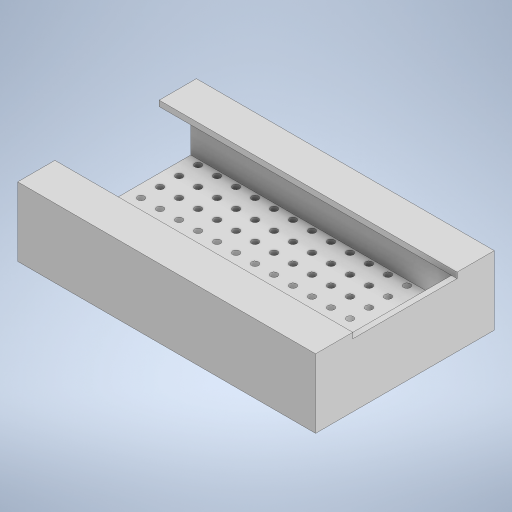
# Autodesk Inventor part: support batterie
Saved by Autodesk Inventor 2024 (Build 280153000, 153)
## iProperties
Created: 2024-02-10
Part Number: support batterie
Material: Generic
Document SubType Name: Modeling
Designer: Pooo
Density: 1 g/cm^3
Appearance: Default
Author: Pooo
Autodesk Inventor part; units mm, degrees
ref_plane "YZ Plane" through (0, 0, 0) normal (1, 0, 0) x (0, 1, 0)
ref_plane "XZ Plane" through (0, 0, 0) normal (0, 1, 0) x (-1, 0, 0)
ref_plane "XY Plane" through (0, 0, 0) normal (0, 0, 1) x (1, 0, 0)
sketch "Sketch1" plane through (0, 0, 0) normal (0, 1, 0) x (-1, 0, 0)
  point P0 (0, 0)
sketch "Sketch2" plane through (0, 0, 0) normal (0, 1, 0) x (-1, 0, 0)
  line L0 (43.1586, 43.7586) -> (-113.8414, 43.7586)
  line L1 (-113.8414, 43.7586) -> (-113.8414, -46.2414)
  line L2 (-113.8414, -46.2414) -> (43.1586, -46.2414)
  line L3 (43.1586, -46.2414) -> (43.1586, 43.7586)
  line L4 (43.1586, -46.2414) -> (-113.8414, -46.2414)
  line L5 (-113.8414, -46.2414) -> (-113.8414, -49.2414)
  line L6 (-113.8414, -49.2414) -> (43.1586, -49.2414)
  line L7 (43.1586, -49.2414) -> (43.1586, -46.2414)
  line L8 (43.1586, 43.7586) -> (-113.8414, 43.7586)
  line L9 (-113.8414, 43.7586) -> (-113.8414, 46.7586)
  line L10 (-113.8414, 46.7586) -> (43.1586, 46.7586)
  line L11 (43.1586, 46.7586) -> (43.1586, 43.7586)
  line L12 (-113.8414, 46.7586) -> (-116.8414, 46.7586)
  line L13 (-116.8414, 46.7586) -> (-116.8414, -49.2414)
  line L14 (-116.8414, -49.2414) -> (-113.8414, -49.2414)
  line L15 (-113.8414, -49.2414) -> (-113.8414, 46.7586)
  point P0 (0, 0)
  dimension "d0" = 90
  dimension "d1" = 157
  dimension "d2" = 3
  dimension "d3" = 3
  dimension "d4" = 3
  constraints: 32 end point, 8 parallel, 4 horizontal, 4 perpendicular
  measures "d0" distance of L2.end L0.start
  measures "d1" distance of L1.end L2.end
  measures "d2" distance of L4.end L5.end
  measures "d3" distance of L8.end L9.end
  measures "d4" distance of L14.end L13.end
extrude "Extrusion1" add sketch "Sketch2" along normal blind 3
sketch "Sketch3" plane through (0, 3, 0) normal (0, 1, 0) x (1, 0, 0)
  line L0 (-43.1586, -46.7586) -> (116.8414, -46.7586) projected
  line L1 (116.8414, -46.7586) -> (116.8414, 49.2414) projected
  line L2 (-43.1586, -46.7586) -> (116.8414, -46.7586)
  line L3 (116.8414, -46.7586) -> (116.8414, -43.7586)
  line L4 (116.8414, -43.7586) -> (-43.1586, -43.7586)
  line L5 (-43.1586, -43.7586) -> (-43.1586, -46.7586)
  line L6 (116.8414, 49.2414) -> (-43.1586, 49.2414) projected
  line L7 (-43.1586, 49.2414) -> (116.8414, 49.2414)
  line L8 (116.8414, 49.2414) -> (116.8414, 46.2414)
  line L9 (116.8414, 46.2414) -> (-43.1586, 46.2414)
  line L10 (-43.1586, 46.2414) -> (-43.1586, 49.2414)
  line L11 (116.8414, -43.7586) -> (113.8414, -43.7586)
  line L12 (113.8414, -43.7586) -> (113.8414, 46.2414)
  line L13 (113.8414, 46.2414) -> (116.8414, 46.2414)
  line L14 (116.8414, 46.2414) -> (116.8414, -43.7586)
  point P0 (0, 0)
  dimension "d7" = 3
  dimension "d8" = 3
  dimension "d9" = 3
  constraints: 24 end point, 6 parallel, 3 horizontal, 3 perpendicular, 3 point on line
  measures "d7" distance of L3.end L2.end
  measures "d8" distance of L7.end L8.end
  measures "d9" distance of L12.end L13.end
sketch "Sketch5" plane through (0, 3, 0) normal (0, 1, 0) x (1, 0, 0)
  circle A0 centre (-36.5125, -38.1) radius 1.85
  line L0 (-36.5125, -38.1) -> (-35.8777, -38.1)
  line L1 (-36.5125, -38.1) -> (-36.5125, -37.4601)
  circle A1 centre (-36.5125, -27.9) radius 1.85
  circle A2 centre (-36.5125, -17.7) radius 1.85
  circle A3 centre (-36.5125, -7.5) radius 1.85
  circle A4 centre (-36.5125, 2.7) radius 1.85
  circle A5 centre (-36.5125, 12.9) radius 1.85
  circle A6 centre (-36.5125, 23.1) radius 1.85
  circle A7 centre (-36.5125, 33.3) radius 1.85
  circle A8 centre (-36.5125, 43.5) radius 1.85
  circle A9 centre (-26.3125, -38.1) radius 1.85
  circle A10 centre (-26.3125, -27.9) radius 1.85
  circle A11 centre (-26.3125, -17.7) radius 1.85
  circle A12 centre (-26.3125, -7.5) radius 1.85
  circle A13 centre (-26.3125, 2.7) radius 1.85
  circle A14 centre (-26.3125, 12.9) radius 1.85
  circle A15 centre (-26.3125, 23.1) radius 1.85
  circle A16 centre (-26.3125, 33.3) radius 1.85
  circle A17 centre (-26.3125, 43.5) radius 1.85
  circle A18 centre (-16.1125, -38.1) radius 1.85
  circle A19 centre (-16.1125, -27.9) radius 1.85
  circle A20 centre (-16.1125, -17.7) radius 1.85
  circle A21 centre (-16.1125, -7.5) radius 1.85
  circle A22 centre (-16.1125, 2.7) radius 1.85
  circle A23 centre (-16.1125, 12.9) radius 1.85
  circle A24 centre (-16.1125, 23.1) radius 1.85
  circle A25 centre (-16.1125, 33.3) radius 1.85
  circle A26 centre (-16.1125, 43.5) radius 1.85
  circle A27 centre (-5.9125, -38.1) radius 1.85
  circle A28 centre (-5.9125, -27.9) radius 1.85
  circle A29 centre (-5.9125, -17.7) radius 1.85
  circle A30 centre (-5.9125, -7.5) radius 1.85
  circle A31 centre (-5.9125, 2.7) radius 1.85
  circle A32 centre (-5.9125, 12.9) radius 1.85
  circle A33 centre (-5.9125, 23.1) radius 1.85
  circle A34 centre (-5.9125, 33.3) radius 1.85
  circle A35 centre (-5.9125, 43.5) radius 1.85
  circle A36 centre (4.2875, -38.1) radius 1.85
  circle A37 centre (4.2875, -27.9) radius 1.85
  circle A38 centre (4.2875, -17.7) radius 1.85
  circle A39 centre (4.2875, -7.5) radius 1.85
  circle A40 centre (4.2875, 2.7) radius 1.85
  circle A41 centre (4.2875, 12.9) radius 1.85
  circle A42 centre (4.2875, 23.1) radius 1.85
  circle A43 centre (4.2875, 33.3) radius 1.85
  circle A44 centre (4.2875, 43.5) radius 1.85
  circle A45 centre (14.4875, -38.1) radius 1.85
  circle A46 centre (14.4875, -27.9) radius 1.85
  circle A47 centre (14.4875, -17.7) radius 1.85
  circle A48 centre (14.4875, -7.5) radius 1.85
  circle A49 centre (14.4875, 2.7) radius 1.85
  circle A50 centre (14.4875, 12.9) radius 1.85
  circle A51 centre (14.4875, 23.1) radius 1.85
  circle A52 centre (14.4875, 33.3) radius 1.85
  circle A53 centre (14.4875, 43.5) radius 1.85
  circle A54 centre (24.6875, -38.1) radius 1.85
  circle A55 centre (24.6875, -27.9) radius 1.85
  circle A56 centre (24.6875, -17.7) radius 1.85
  circle A57 centre (24.6875, -7.5) radius 1.85
  circle A58 centre (24.6875, 2.7) radius 1.85
  circle A59 centre (24.6875, 12.9) radius 1.85
  circle A60 centre (24.6875, 23.1) radius 1.85
  circle A61 centre (24.6875, 33.3) radius 1.85
  circle A62 centre (24.6875, 43.5) radius 1.85
  circle A63 centre (34.8875, -38.1) radius 1.85
  circle A64 centre (34.8875, -27.9) radius 1.85
  circle A65 centre (34.8875, -17.7) radius 1.85
  circle A66 centre (34.8875, -7.5) radius 1.85
  circle A67 centre (34.8875, 2.7) radius 1.85
  circle A68 centre (34.8875, 12.9) radius 1.85
  circle A69 centre (34.8875, 23.1) radius 1.85
  circle A70 centre (34.8875, 33.3) radius 1.85
  circle A71 centre (34.8875, 43.5) radius 1.85
  circle A72 centre (45.0875, -38.1) radius 1.85
  circle A73 centre (45.0875, -27.9) radius 1.85
  circle A74 centre (45.0875, -17.7) radius 1.85
  circle A75 centre (45.0875, -7.5) radius 1.85
  circle A76 centre (45.0875, 2.7) radius 1.85
  circle A77 centre (45.0875, 12.9) radius 1.85
  circle A78 centre (45.0875, 23.1) radius 1.85
  circle A79 centre (45.0875, 33.3) radius 1.85
  circle A80 centre (45.0875, 43.5) radius 1.85
  circle A81 centre (55.2875, -38.1) radius 1.85
  circle A82 centre (55.2875, -27.9) radius 1.85
  circle A83 centre (55.2875, -17.7) radius 1.85
  circle A84 centre (55.2875, -7.5) radius 1.85
  circle A85 centre (55.2875, 2.7) radius 1.85
  circle A86 centre (55.2875, 12.9) radius 1.85
  circle A87 centre (55.2875, 23.1) radius 1.85
  circle A88 centre (55.2875, 33.3) radius 1.85
  circle A89 centre (55.2875, 43.5) radius 1.85
  circle A90 centre (65.4875, -38.1) radius 1.85
  circle A91 centre (65.4875, -27.9) radius 1.85
  circle A92 centre (65.4875, -17.7) radius 1.85
  circle A93 centre (65.4875, -7.5) radius 1.85
  circle A94 centre (65.4875, 2.7) radius 1.85
  circle A95 centre (65.4875, 12.9) radius 1.85
  circle A96 centre (65.4875, 23.1) radius 1.85
  circle A97 centre (65.4875, 33.3) radius 1.85
  circle A98 centre (65.4875, 43.5) radius 1.85
  circle A99 centre (75.6875, -38.1) radius 1.85
  circle A100 centre (75.6875, -27.9) radius 1.85
  circle A101 centre (75.6875, -17.7) radius 1.85
  circle A102 centre (75.6875, -7.5) radius 1.85
  circle A103 centre (75.6875, 2.7) radius 1.85
  circle A104 centre (75.6875, 12.9) radius 1.85
  circle A105 centre (75.6875, 23.1) radius 1.85
  circle A106 centre (75.6875, 33.3) radius 1.85
  circle A107 centre (75.6875, 43.5) radius 1.85
  circle A108 centre (85.8875, -38.1) radius 1.85
  circle A109 centre (85.8875, -27.9) radius 1.85
  circle A110 centre (85.8875, -17.7) radius 1.85
  circle A111 centre (85.8875, -7.5) radius 1.85
  circle A112 centre (85.8875, 2.7) radius 1.85
  circle A113 centre (85.8875, 12.9) radius 1.85
  circle A114 centre (85.8875, 23.1) radius 1.85
  circle A115 centre (85.8875, 33.3) radius 1.85
  circle A116 centre (85.8875, 43.5) radius 1.85
  circle A117 centre (96.0875, -38.1) radius 1.85
  circle A118 centre (96.0875, -27.9) radius 1.85
  circle A119 centre (96.0875, -17.7) radius 1.85
  circle A120 centre (96.0875, -7.5) radius 1.85
  circle A121 centre (96.0875, 2.7) radius 1.85
  circle A122 centre (96.0875, 12.9) radius 1.85
  circle A123 centre (96.0875, 23.1) radius 1.85
  circle A124 centre (96.0875, 33.3) radius 1.85
  circle A125 centre (96.0875, 43.5) radius 1.85
  circle A126 centre (106.2875, -38.1) radius 1.85
  circle A127 centre (106.2875, -27.9) radius 1.85
  circle A128 centre (106.2875, -17.7) radius 1.85
  circle A129 centre (106.2875, -7.5) radius 1.85
  circle A130 centre (106.2875, 2.7) radius 1.85
  circle A131 centre (106.2875, 12.9) radius 1.85
  circle A132 centre (106.2875, 23.1) radius 1.85
  circle A133 centre (106.2875, 33.3) radius 1.85
  circle A134 centre (106.2875, 43.5) radius 1.85
  point P0 (0, 0)
  dimension "d10" = 3.7
  dimension "d13" = 10.2
  dimension "d16" = 10.2
  constraints: 135 centre point, 4 end point, 2 horizontal, 2 vertical, 268 other
  measures "d10" diameter of A0
  measures "d13" distance of L0.start A1.centre
  measures "d16" distance of L0.start A9.centre
extrude "Extrusion2" cut sketch "Sketch5" against normal blind 4
extrude "Extrusion3" add sketch "Sketch3" along normal blind 31
sketch "Sketch8" plane through (0, 34, 0) normal (0, 1, 0) x (1, 0, 0)
  line L0 (116.8414, -46.7586) -> (116.8414, 49.2414) projected
  line L1 (-43.1586, 49.2414) -> (116.8414, 49.2414)
  line L2 (116.8414, 49.2414) -> (116.8414, 29.2414)
  line L3 (116.8414, 29.2414) -> (-43.1586, 29.2414)
  line L4 (-43.1586, 29.2414) -> (-43.1586, 49.2414)
  line L5 (116.8414, -46.7586) -> (-43.1586, -46.7586)
  line L6 (-43.1586, -46.7586) -> (-43.1586, -26.7586)
  line L7 (-43.1586, -26.7586) -> (116.8414, -26.7586)
  line L8 (116.8414, -26.7586) -> (116.8414, -46.7586)
  point P0 (0, 0)
  dimension "d23" = 20
  dimension "d24" = 20
  constraints: 16 end point, 4 parallel, 2 horizontal, 2 perpendicular, 2 point on line
  measures "d23" distance of L1.end L2.end
  measures "d24" distance of L5.end L6.end
extrude "Extrusion4" add sketch "Sketch8" along normal blind 3
body "Solid1"
